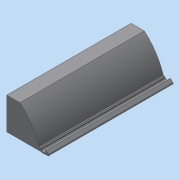
# Autodesk Inventor part: 0 零件
Saved by Autodesk Inventor 2020 (Build 240168000, 168)
## iProperties
Created: 2020-11-03
Part Number: 0 零件
Material: 一般
Document SubType Name: Modeling
Designer: p2013
Density: 1 g/cm^3
Appearance: 預設
Author: p2013
Autodesk Inventor part; units mm, degrees
ref_plane "YZ Plane" through (0, 0, 0) normal (1, 0, 0) x (0, 1, 0)
ref_plane "XZ Plane" through (0, 0, 0) normal (0, 1, 0) x (-1, 0, 0)
ref_plane "XY Plane" through (0, 0, 0) normal (0, 0, 1) x (1, 0, 0)
sketch "草圖3" plane through (0, 0, 0) normal (0, 1, 0) x (-1, 0, 0)
  line L0 (0, 0) -> (0, -300)
  dimension "d15" = 300
  constraints: 2 end point, 1 vertical
  measures "d15" distance of L0.start L0.end
sketch "草圖1" plane through (0, 0, 0) normal (0, 0, 1) x (1, 0, 0)
  line L0 (0, 0) -> (-9.6483, 0) construction
  line L1 (0, 0) -> (0, 9.3404) construction
  line L2 (-8.1216, 4.6307) -> (-8.4962, 8.9128)
  arc A0 (-6.8323, 9.7444) -> (-8.4962, 8.9128) centre (-7.5, 9) ccw
  line L3 (-6.8323, 9.7444) -> (-0.8307, 4.361)
  arc A1 (-4.5, 1) -> (-0.8307, 4.361) centre (-2.5, 2.5) ccw
  line L4 (-4.5, 1) -> (-6, 1)
  line L5 (-6, 1) -> (-8, 0)
  line L6 (-8, 0) -> (-15.9689, 0)
  line L7 (-15.9689, 0) -> (-18.1528, 1)
  line L8 (-18.1528, 1) -> (-101.5326, 1)
  line L9 (-9.6159, 3) -> (-17.1685, 3)
  arc A2 (-9.6159, 3) -> (-8.1216, 4.6307) centre (-9.6159, 4.5) ccw
  line L10 (-19.1004, 4.4824) -> (-19.5385, 6.1176)
  line L11 (-21.4704, 7.5999) -> (-22.2327, 7.5999)
  arc A3 (-19.5385, 6.1176) -> (-21.4704, 7.5999) centre (-21.4704, 5.5999) ccw
  arc A4 (-19.1004, 4.4824) -> (-17.1685, 3) centre (-17.1685, 5) ccw
  line L12 (-14, 16.4786) -> (-11, 16.4786) construction
  line L13 (-11, 16.4786) -> (-11, 4.7787) construction
  line L14 (-11, 4.7787) -> (-14, 4.7787) construction
  line L15 (-14, 4.7787) -> (-14, 16.4786) construction
  arc A5 (-24.139, 8.995) -> (-69.7556, 77.7407) centre (-167.1146, -36.3699) ccw
  arc A6 (-24.139, 8.995) -> (-22.2327, 7.5999) centre (-22.2327, 9.5999) ccw
  line L16 (-69.7556, 77.7407) -> (-101.5326, 77.7407)
  line L17 (-101.5326, 77.7407) -> (-101.5326, 1)
  point P0 (-23.7038, 7.5999)
  point P1 (-12.5, 4.7787)
  dimension "d0" = 10
  dimension "d4" = 1
  dimension "d5" = 2.5
  dimension "d8" = 1.5
  dimension "d9" = 2
  dimension "d10" = 2
  dimension "d11" = 105
  dimension "d13" = 3
  dimension "d14" = 10
  dimension "d20" = 5
  dimension "d21" = 85
  dimension "d22" = 3
  dimension "d24" = 150
  dimension "d25" = 2
  dimension "d26" = 2
  dimension "d27" = 7.9689
  dimension "d28" = 2
  dimension "d29" = 1.5
  constraints: 36 end point, 15 point on circle, 13 tangent, 7 centre point, 6 horizontal, 4 point on line, 3 parallel, 2 perpendicular, 1 midpoint, 1 vertical
  measures "d4" radius of A0
  measures "d5" radius of A1
  measures "d8" radius of A2
  measures "d9" radius of A3
  measures "d10" radius of A4
  measures "d11" angle of L9 L10
  measures "d13" distance of L12.start L12.end
  measures "d14" horizontal distance of A1.centre point (-12.5, 4.779)
  measures "d20" horizontal distance of A0.centre A1.centre
  measures "d21" angle of L9 L2
  measures "d22" distance between parallel lines of L6 L9
  measures "d24" radius of A5
  measures "d25" radius of A6
  measures "d26" distance between parallel lines of L9 L8
  measures "d27" distance of L5.end L6.end
  measures "d28" horizontal distance of L4.end L5.end
  measures "d29" distance of L4.start L4.end
sweep "掃掠1" add profiles "草圖1" path "草圖3"
fillet "圓角1" radius 2 3 edges at (-6, 1, -150) (-4.5, 1, -150) (-8, 0, -150)
